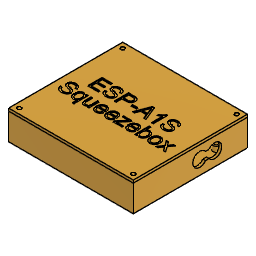
SqueezeboxCase (Autodesk Fusion 360 design; units mm, degrees)
Autodesk Fusion 360 part; units mm, degrees
sketch "Sketch1" plane through (0, 0, 0) normal (0, 0, 1) x (1, 0, 0)
  line L0 (-86.1759, 61.7908) -> (-4.1759, 61.7908)
  line L1 (-4.1759, 61.7908) -> (-4.1759, -12.2092)
  line L2 (-4.1759, -12.2092) -> (-86.1759, -12.2092)
  line L3 (-86.1759, -12.2092) -> (-86.1759, 61.7908)
  line L4 (-0.1759, -16.2092) -> (-90.1759, -16.2092)
  line L5 (-90.1759, -16.2092) -> (-90.1759, 65.7908)
  line L6 (-90.1759, 65.7908) -> (-0.1759, 65.7908)
  line L7 (-0.1759, 65.7908) -> (-0.1759, -16.2092)
  line L8 (1.8241, -18.2092) -> (-92.1759, -18.2092)
  line L9 (-92.1759, -18.2092) -> (-92.1759, 67.7908)
  line L10 (-92.1759, 67.7908) -> (1.8241, 67.7908)
  line L11 (1.8241, 67.7908) -> (1.8241, -18.2092)
  line L12 (-86.1759, 61.7908) -> (-82.6759, 61.7908)
  line L13 (-86.1759, 58.2908) -> (-86.1759, 61.7908)
  line L14 (-86.1759, -12.2092) -> (-82.6759, -12.2092)
  line L15 (-82.6759, -12.2092) -> (-82.6759, -8.7092)
  line L16 (-82.6759, -8.7092) -> (-86.1759, -8.7092)
  line L17 (-86.1759, -8.7092) -> (-86.1759, -12.2092)
  line L18 (-4.1759, -12.2092) -> (-7.6759, -12.2092)
  line L19 (-7.6759, -12.2092) -> (-7.6759, -8.7092)
  line L20 (-7.6759, -8.7092) -> (-4.1759, -8.7092)
  line L21 (-4.1759, -8.7092) -> (-4.1759, -12.2092)
  circle A0 centre (-82.6759, -8.7092) radius 1.1
  circle A1 centre (-7.6759, -8.7092) radius 1.1
  line L22 (-86.1759, 61.7908) -> (-3.1759, 61.7908)
  line L23 (-3.1759, 61.7908) -> (-3.1759, 56.2908)
  line L24 (-3.1759, 56.2908) -> (-86.1759, 56.2908)
  line L25 (-86.1759, 56.2908) -> (-86.1759, 61.7908)
  line L26 (-86.1759, 56.2908) -> (-82.6759, 56.2908)
  line L27 (-82.6759, 56.2908) -> (-82.6759, 52.7908)
  line L28 (-82.6759, 52.7908) -> (-86.1759, 52.7908)
  line L29 (-86.1759, 52.7908) -> (-86.1759, 56.2908)
  line L30 (-3.1759, 56.2908) -> (-6.6759, 56.2908)
  line L31 (-6.6759, 56.2908) -> (-6.6759, 52.7908)
  line L32 (-6.6759, 52.7908) -> (-3.1759, 52.7908)
  line L33 (-3.1759, 52.7908) -> (-3.1759, 56.2908)
  circle A2 centre (-6.6759, 52.7908) radius 1.1
  circle A3 centre (-82.6759, 52.7908) radius 1.1
  circle A4 centre (-6.6759, 52.7908) radius 2.4
  circle A5 centre (-82.6759, 52.7908) radius 2.4
  circle A6 centre (-82.6759, -8.7092) radius 2.4
  circle A7 centre (-7.6759, -8.7092) radius 2.4
  line L34 (-90.1759, 65.7908) -> (-86.1759, 65.7908)
  line L35 (-86.1759, 65.7908) -> (-86.1759, 61.7908)
  line L36 (-86.1759, 61.7908) -> (-90.1759, 61.7908)
  line L37 (-90.1759, 61.7908) -> (-90.1759, 65.7908)
  line L38 (-0.1759, 65.7908) -> (-4.1759, 65.7908)
  line L39 (-4.1759, 65.7908) -> (-4.1759, 61.7908)
  line L40 (-4.1759, 61.7908) -> (-0.1759, 61.7908)
  line L41 (-0.1759, 61.7908) -> (-0.1759, 65.7908)
  line L42 (-0.1759, -16.2092) -> (-4.1759, -16.2092)
  line L43 (-4.1759, -16.2092) -> (-4.1759, -12.2092)
  line L44 (-4.1759, -12.2092) -> (-0.1759, -12.2092)
  line L45 (-0.1759, -12.2092) -> (-0.1759, -16.2092)
  line L46 (-90.1759, -16.2092) -> (-86.1759, -16.2092)
  line L47 (-86.1759, -16.2092) -> (-86.1759, -12.2092)
  line L48 (-86.1759, -12.2092) -> (-90.1759, -12.2092)
  line L49 (-90.1759, -12.2092) -> (-90.1759, -16.2092)
  circle A8 centre (-88.1759, 63.7908) radius 1.25
  circle A9 centre (-2.1759, 63.7908) radius 1.25
  circle A10 centre (-2.1759, -14.2092) radius 1.25
  circle A11 centre (-88.1759, -14.2092) radius 1.25
  circle A12 centre (-88.1759, 63.7908) radius 1.55
  circle A13 centre (-2.1759, 63.7908) radius 1.55
  circle A14 centre (-2.1759, -14.2092) radius 1.55
  circle A15 centre (-88.1759, -14.2092) radius 1.55
  point P0 (-2.1759, 63.7908)
  point P1 (-2.1759, -14.2092)
  dimension "d1" = 82
  dimension "d2" = 74
  dimension "d3" = -4
  dimension "d4" = -6
  dimension "d8" = 3.5
  dimension "d9" = 3.5
  dimension "d10" = 3.5
  dimension "d11" = 3.5
  dimension "d12" = 2.2
  dimension "d13" = 2.2
  dimension "d14" = 5.5
  dimension "d15" = 3.5
  dimension "d16" = 3.5
  dimension "d17" = 3.5
  dimension "d18" = 3.5
  dimension "d19" = 2.2
  dimension "d20" = 2.2
  dimension "d27" = 1.3
  dimension "d28" = 1.3
  dimension "d29" = 1.3
  dimension "d30" = 1.3
  dimension "d61" = 2.5
  dimension "d62" = 2.5
  dimension "d63" = 2.5
  dimension "d64" = 2.5
  dimension "d67" = 0.3
  dimension "d68" = 0.3
  dimension "d69" = 0.3
  dimension "d70" = 0.3
  constraint horizontal L0
  constraint vertical L1
  constraint horizontal L2
  constraint vertical L3
  constraint horizontal L12
  constraint vertical L13
  constraint horizontal L14
  constraint vertical L15
  constraint horizontal L16
  constraint vertical L17
  constraint horizontal L18
  constraint vertical L19
  constraint horizontal L20
  constraint vertical L21
  constraint coincident L15.end L16.start
  constraint coincident L19.end L20.start
  constraint horizontal L22
  constraint vertical L23
  constraint horizontal L24
  constraint vertical L25
  constraint horizontal L26
  constraint vertical L27
  constraint horizontal L28
  constraint vertical L29
  constraint horizontal L30
  constraint vertical L31
  constraint horizontal L32
  constraint vertical L33
  constraint coincident L31.end L32.start
  constraint coincident L27.end L28.start
  constraint horizontal L34
  constraint vertical L35
  constraint horizontal L36
  constraint vertical L37
  constraint horizontal L38
  constraint vertical L39
  constraint horizontal L40
  constraint vertical L41
  constraint horizontal L42
  constraint vertical L43
  constraint horizontal L44
  constraint vertical L45
  constraint horizontal L46
  constraint vertical L47
  constraint horizontal L48
  constraint vertical L49
  constraint coincident P0 A9.centre
  constraint coincident P1 A10.centre
  measures "d1" distance of L0.start L0.end
  measures "d2" distance of L0.start L2.end
  measures "d8" distance of L2.end L14.end
  measures "d9" distance of L2.end L16.end
  measures "d10" distance of L1.end L18.end
  measures "d11" distance of L1.end L20.end
  measures "d12" diameter of A0
  measures "d13" diameter of A1
  measures "d14" distance of L0.start L24.end
  measures "d15" distance of L24.end L26.end
  measures "d16" distance of L24.end L28.end
  measures "d17" distance of L23.end L30.end
  measures "d18" distance of L23.end L32.end
  measures "d19" diameter of A2
  measures "d20" diameter of A3
  measures "d61" diameter of A8
  measures "d62" diameter of A9
  measures "d63" diameter of A10
  measures "d64" diameter of A11
extrude "Extrude1" add sketch "Sketch1" against normal blind 2 contours L0 L6 L12 L22 L35 L39 | L0 L1 L3 L12 L13 L22 L24 L25 L26 L30 | L5 L6 L34 L35 L36 L37 | L3 L5 L13 L17 L25 L29 L36 L48 | L1 L22 L23 L24 L30 L40 | L6 L7 L22 L38 L39 L40 L41 | L3 L24 L26 L27 L28 L29 A5 | L4 L5 L46 L47 L48 L49 | L1 L24 L30 L32 L33 | L1 L24 L30 L31 L32 A4 | L1 L7 L21 L23 L32 L33 L40 L44 | L1 L2 L3 L15 L16 L19 L20 L24 L27 L28 L31 L32 A4 A5 A6 A7 | L2 L3 L14 L15 L16 L17 A6 | L2 L4 L14 L18 L43 L47 | L27 L28 A3 A5 | L27 L28 A3 A5 | L1 L2 L18 L19 L20 L21 A7 | L31 L32 A2 A4 | L31 L32 A2 A4 | L4 L7 L42 L43 L44 L45 | L15 L16 A0 A6 | L15 L16 A0 A6 | L27 L28 A3 | L27 L28 A3 | L19 L20 A1 A7 | L19 L20 A1 A7 | L31 L32 A2 | L31 L32 A2 | L15 L16 A0 | L15 L16 A0 | L19 L20 A1 | L19 L20 A1 | L8 L9 L10 L11 | A8 | A9 | A10 | A11 | A12 | A13 | A14 | A15 makes body 1
extrude "Extrude2" add sketch "Sketch1" along normal blind 18 contours L8 L9 L10 L11 bodies 1
extrude "Extrude3" add sketch "Sketch1" along normal blind 8 contours L27 L28 A3 | L27 L28 A3 | L31 L32 A2 | L31 L32 A2 | L15 L16 A0 | L15 L16 A0 | L19 L20 A1 | L19 L20 A1 bodies 1
extrude "Extrude4" add sketch "Sketch1" along normal blind 4 contours L27 L28 A3 A5 | L27 L28 A3 A5 | L31 L32 A2 A4 | L31 L32 A2 A4 | L15 L16 A0 A6 | L15 L16 A0 A6 | L19 L20 A1 A7 | L19 L20 A1 A7 bodies 1
sketch "Sketch2" plane through (1.8241, 0, 0) normal (1, 0, 0) x (0, 1, 0)
  line L0 (-18.2092, 18) -> (-18.2092, -2)
  line L1 (-18.2092, -2) -> (67.7908, -2)
  line L2 (67.7908, -2) -> (67.7908, 18)
  line L3 (67.7908, 18) -> (-18.2092, 18)
  line L4 (67.7908, -2) -> (-18.2092, -2)
  line L5 (-18.2092, -2) -> (-18.2092, 5.5)
  line L6 (-18.2092, 5.5) -> (67.7908, 5.5)
  line L7 (67.7908, 5.5) -> (67.7908, -2)
  line L8 (67.7908, 5.5) -> (46.7908, 5.5)
  line L9 (46.7908, 5.5) -> (46.7908, 11.5)
  line L10 (46.7908, 11.5) -> (67.7908, 11.5)
  line L11 (67.7908, 11.5) -> (67.7908, 5.5)
  line L12 (46.7908, 11.5) -> (28.2908, 11.5)
  line L13 (28.2908, 11.5) -> (28.2908, 5.5)
  line L14 (28.2908, 5.5) -> (46.7908, 5.5)
  line L15 (46.7908, 5.5) -> (46.7908, 11.5)
  line L16 (28.2908, 11.5) -> (31.8908, 11.5)
  line L17 (31.8908, 11.5) -> (31.8908, 5.5)
  line L18 (31.8908, 5.5) -> (28.2908, 5.5)
  line L19 (28.2908, 5.5) -> (28.2908, 11.5)
  line L20 (46.7908, 11.5) -> (43.1908, 11.5)
  line L21 (43.1908, 11.5) -> (43.1908, 5.5)
  line L22 (43.1908, 5.5) -> (46.7908, 5.5)
  line L23 (46.7908, 5.5) -> (46.7908, 11.5)
  circle A0 centre (31.8908, 8.5) radius 5.25
  circle A1 centre (43.1908, 8.5) radius 5.25
  dimension "d33" = 86
  dimension "d34" = 7.5
  dimension "d35" = 21
  dimension "d36" = 6
  dimension "d37" = 18.5
  dimension "d38" = 6
  dimension "d71" = 6
  dimension "d72" = 3.6
  dimension "d73" = 6
  dimension "d74" = 3.6
  dimension "d75" = 10.5
  dimension "d76" = 10.5
  constraint horizontal L4
  constraint vertical L5
  constraint horizontal L6
  constraint vertical L7
  constraint coincident L1.end L2.start
  constraint horizontal L8
  constraint vertical L9
  constraint horizontal L10
  constraint vertical L11
  constraint horizontal L12
  constraint vertical L13
  constraint horizontal L14
  constraint vertical L15
  constraint horizontal L16
  constraint vertical L17
  constraint horizontal L18
  constraint vertical L19
  constraint horizontal L20
  constraint vertical L21
  constraint horizontal L22
  constraint vertical L23
  constraint midpoint L17 A0.centre
  constraint midpoint L21 A1.centre
  measures "d33" distance of L1.end L0.end
  measures "d34" distance of L1.end L6.end
  measures "d35" distance of L6.end L8.end
  measures "d36" distance of L6.end L10.end
  measures "d37" distance of L9.end L12.end
  measures "d38" distance of L9.end L8.end
  measures "d71" distance of L12.end L13.end
  measures "d72" distance of L12.end L16.end
  measures "d73" distance of L9.end L8.end
  measures "d74" distance of L9.end L20.end
  measures "d75" diameter of A0
  measures "d76" diameter of A1
extrude "Extrude5" cut sketch "Sketch2" against normal up to surface (2 mm away) contours L6 L12 L13 L16 L19 A0 | L6 L14 L18 A0 | L6 L12 L13 L14 L16 L17 L18 L19 | L6 L12 L14 L17 A0 | L6 L12 L14 A0 A1 | L6 L8 L9 L10 L15 L23 A1 | L10 L12 L20 A1 | L6 L12 L14 L21 A1 | L6 L8 L14 L22 A1 | L6 L9 L12 L14 L15 L20 L21 L22 L23 bodies 1
sketch "Sketch3" plane through (-92.1759, 0, 0) normal (-1, 0, 0) x (0, -1, 0)
  line L0 (-67.7908, 18) -> (-67.7908, -2)
  line L1 (-67.7908, -2) -> (18.2092, -2)
  line L2 (18.2092, -2) -> (18.2092, 18)
  line L3 (18.2092, 18) -> (-67.7908, 18)
  line L4 (-67.7908, -2) -> (18.2092, -2)
  line L5 (18.2092, -2) -> (18.2092, 3.5)
  line L6 (18.2092, 3.5) -> (-67.7908, 3.5)
  line L7 (-67.7908, 3.5) -> (-67.7908, -2)
  line L8 (-67.7908, 3.5) -> (-56.2908, 3.5)
  line L9 (-56.2908, 3.5) -> (-56.2908, 11.5)
  line L10 (-56.2908, 11.5) -> (-67.7908, 11.5)
  line L11 (-67.7908, 11.5) -> (-67.7908, 3.5)
  line L12 (-56.2908, 11.5) -> (-17.2908, 11.5)
  line L13 (-17.2908, 11.5) -> (-17.2908, 2.3145)
  line L14 (-56.2908, 2.3145) -> (-56.2908, 11.5)
  line L15 (-17.2908, 11.5) -> (-5.2908, 11.5)
  line L16 (-5.2908, 11.5) -> (-5.2908, 3.5)
  line L17 (-5.2908, 3.5) -> (-17.2908, 3.5)
  line L18 (-17.2908, 3.5) -> (-17.2908, 11.5)
  dimension "d41" = 5.5
  dimension "d42" = 11.5
  dimension "d43" = 8
  dimension "d45" = 39
  dimension "d46" = 12
  constraint horizontal L4
  constraint vertical L5
  constraint horizontal L6
  constraint vertical L7
  constraint coincident L0.end L1.start
  constraint horizontal L8
  constraint vertical L9
  constraint horizontal L10
  constraint vertical L11
  constraint horizontal L12
  constraint vertical L13
  constraint vertical L14
  constraint horizontal L15
  constraint vertical L16
  constraint horizontal L17
  constraint vertical L18
  constraint collinear L6 L17
  measures "d41" distance of L0.end L6.end
  measures "d42" distance of L6.end L8.end
  measures "d43" distance of L6.end L10.end
  measures "d45" distance of L9.end L12.end
  measures "d46" distance of L12.end L15.end
extrude "Extrude6" cut sketch "Sketch3" against normal up to surface (2 mm away) contours L6 L13 L15 L16 L17 L18 bodies 1
extrude "Extrude7" add sketch "Sketch1" against normal blind 2 separate body contours L0 L6 L12 L22 L35 L39 | L0 L1 L3 L12 L13 L22 L24 L25 L26 L30 | L5 L6 L34 L35 L36 L37 | L3 L5 L13 L17 L25 L29 L36 L48 | L1 L22 L23 L24 L30 L40 | L6 L7 L22 L38 L39 L40 L41 | L3 L24 L26 L27 L28 L29 A5 | L4 L5 L46 L47 L48 L49 | L1 L24 L30 L32 L33 | L1 L24 L30 L31 L32 A4 | L1 L7 L21 L23 L32 L33 L40 L44 | L1 L2 L3 L15 L16 L19 L20 L24 L27 L28 L31 L32 A4 A5 A6 A7 | L2 L3 L14 L15 L16 L17 A6 | L2 L4 L14 L18 L43 L47 | L27 L28 A3 A5 | L27 L28 A3 A5 | L1 L2 L18 L19 L20 L21 A7 | L31 L32 A2 A4 | L31 L32 A2 A4 | L4 L7 L42 L43 L44 L45 | L15 L16 A0 A6 | L15 L16 A0 A6 | L27 L28 A3 | L27 L28 A3 | L19 L20 A1 A7 | L19 L20 A1 A7 | L31 L32 A2 | L31 L32 A2 | L15 L16 A0 | L15 L16 A0 | L19 L20 A1 | L19 L20 A1 | L8 L9 L10 L11 makes body 2
extrude "Extrude8" add sketch "Sketch1" along normal blind 2 contours L0 L6 L12 L22 L35 L39 | L0 L1 L3 L12 L13 L22 L24 L25 L26 L30 | L5 L6 L34 L35 L36 L37 | L3 L5 L13 L17 L25 L29 L36 L48 | L1 L22 L23 L24 L30 L40 | L6 L7 L22 L38 L39 L40 L41 | L3 L24 L26 L27 L28 L29 A5 | L4 L5 L46 L47 L48 L49 | L1 L24 L30 L32 L33 | L1 L24 L30 L31 L32 A4 | L1 L7 L21 L23 L32 L33 L40 L44 | L1 L2 L3 L15 L16 L19 L20 L24 L27 L28 L31 L32 A4 A5 A6 A7 | L2 L3 L14 L15 L16 L17 A6 | L2 L4 L14 L18 L43 L47 | L27 L28 A3 A5 | L27 L28 A3 A5 | L1 L2 L18 L19 L20 L21 A7 | L31 L32 A2 A4 | L31 L32 A2 A4 | L4 L7 L42 L43 L44 L45 | L15 L16 A0 A6 | L15 L16 A0 A6 | L27 L28 A3 | L27 L28 A3 | L19 L20 A1 A7 | L19 L20 A1 A7 | L31 L32 A2 | L31 L32 A2 | L15 L16 A0 | L15 L16 A0 | L19 L20 A1 | L19 L20 A1 bodies 2
fillet "Fillet1" radius 0.5 4 edges at (-0.1759, -16.2092, 1) (-0.1759, 65.7908, 1) (-90.1759, 65.7908, 1) (-90.1759, -16.2092, 1) on bodies 2
move_body "Move1" bodies 2 to x (-1, 0, 0) y (0, 1, 0) z (0, 0, -1) at (-85.3518, 0, 50)
move_body "Move2" bodies 2 to x (1, 0, 0) y (0, 1, 0) z (0, 0, 1) at (-4, 0, 0)
move_body "Move3" bodies 2 to x (1, 0, 0) y (0, 1, 0) z (0, 0, 1) at (0, 0, -32)
sketch "Sketch4" plane through (0, 0, 20) normal (0, 0, 1) x (-1, 0, 0)
  line L0 (-2.8241, -67.7908) -> (91.1759, -67.7908)
  line L1 (91.1759, -67.7908) -> (91.1759, 18.2092)
  line L2 (91.1759, 18.2092) -> (-2.8241, 18.2092)
  line L3 (-2.8241, 18.2092) -> (-2.8241, -67.7908)
  line L4 (85.9929, -9.236) -> (3.3757, -9.236) construction
  line L5 (3.3757, -9.236) -> (3.3757, -24.236) construction
  line L6 (3.3757, -24.236) -> (85.9929, -24.236) construction
  line L7 (85.9929, -24.236) -> (85.9929, -9.236) construction
  line L8 (75.9165, -25.9903) -> (14.5249, -25.9903) construction
  line L9 (14.5249, -25.9903) -> (14.5249, -40.9903) construction
  line L10 (14.5249, -40.9903) -> (75.9165, -40.9903) construction
  line L11 (75.9165, -40.9903) -> (75.9165, -25.9903) construction
  line L12 (91.1759, -67.7908) -> (-3.8241, -67.7908)
  line L13 (-3.8241, -67.7908) -> (-3.8241, -24.7908)
  line L14 (-3.8241, -24.7908) -> (91.1759, -24.7908)
  line L15 (91.1759, -24.7908) -> (91.1759, -67.7908)
  line L16 (91.1759, -67.7908) -> (43.6759, -67.7908)
  line L17 (43.6759, -67.7908) -> (43.6759, 18.2092)
  line L18 (43.6759, 18.2092) -> (91.1759, 18.2092)
  line L19 (91.1759, 18.2092) -> (91.1759, -67.7908)
  circle A0 centre (87.1759, 14.2092) radius 1.55
  circle A1 centre (87.1759, -63.7908) radius 1.55
  circle A2 centre (1.1759, 14.2092) radius 1.55
  circle A3 centre (1.1759, -63.7908) radius 1.55
  dimension "d54" = 95
  dimension "d55" = 43
  dimension "d56" = 47.5
  text T0 "Squeezebox" font "Arial" height 15 align ink ink in box 0 x 0 at (85.9929, -9.236) x (-1, 0) y (0, -1) spacing 1 height is em
  text T1 "ESP-A1S" font "Arial" height 15 align ink ink in box 0 x 0 at (75.9165, -25.9903) x (-1, 0) y (0, -1) spacing 1 height is em
  constraint perpendicular L4 L5
  constraint parallel L4 L6
  constraint parallel L5 L7
  constraint perpendicular L8 L9
  constraint parallel L8 L10
  constraint parallel L9 L11
  constraint horizontal L12
  constraint vertical L13
  constraint horizontal L14
  constraint vertical L15
  constraint coincident L0.end L1.start
  constraint horizontal L16
  constraint vertical L17
  constraint horizontal L18
  constraint vertical L19
  measures "d54" distance of L0.end L12.end
  measures "d55" distance of L0.end L14.end
  measures "d56" distance of L0.end L16.end
extrude "Extrude9" cut sketch "Sketch4" against normal blind 0.5 text T1 T0 bodies 2
extrude "Extrude10" add sketch "Sketch1" along normal blind 16 contours L5 L6 L34 L35 L36 L37 | L6 L7 L22 L38 L39 L40 L41 | L4 L5 L46 L47 L48 L49 | L4 L7 L42 L43 L44 L45 | A8 | A9 | A10 | A11 | A12 | A13 | A14 | A15 bodies 1
extrude "Extrude11" add sketch "Sketch1" along normal up to surface (20 mm away) contours A8 | A9 | A10 | A11 bodies 1
move_body "Move4" bodies 2 to x (1, 0, 0) y (0, 1, 0) z (0, 0, 1) at (-1, 0, 0)
equation "d12 = 2.5 mm - 0.3 mm"
equation "d13 = 2.5 mm - 0.3 mm"
equation "d19 = 2.5 mm - 0.3 mm"
equation "d27 = 1.0000000149 mm + 0.3 mm"
equation "d28 = 1.0000000149 mm + 0.3 mm"
equation "d29 = 1.0000000149 mm + 0.3 mm"
equation "d30 = 1.0000000149 mm + 0.3 mm"
equation "d34 = 3.5 mm + 4 mm"
equation "d35 = 9.5 mm + 11.5 mm"
equation "d41 = 6.5 mm - 1 mm"
equation "d42 = 9.5 mm + 2 mm"
named bodies: "Case", "Top"
